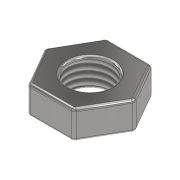
# Autodesk Inventor part: M3_nut
Saved by Autodesk Inventor 2020 (Build 240168000, 168)
## iProperties
Created: 2021-02-03
Part Number: M3_nut
Material: Generic
Document SubType Name: Modeling
Designer: JojoS
Density: 1 g/cm^3
Appearance: Steel - Polished
Author: JojoS
Autodesk Inventor part; units mm, degrees
ref_plane "YZ Plane" through (0, 0, 0) normal (1, 0, 0) x (0, 1, 0)
ref_plane "XZ Plane" through (0, 0, 0) normal (0, 1, 0) x (-1, 0, 0)
ref_plane "XY Plane" through (0, 0, 0) normal (0, 0, 1) x (1, 0, 0)
sketch "Sketch1" plane through (0, 0, 0) normal (0, 1, 0) x (-1, 0, 0)
  circle A0 centre (0, 0) radius 1.65
  line L0 (-1.7609, -3.05) -> (-3.5218, 0)
  line L1 (-3.5218, 0) -> (-1.7609, 3.05)
  line L2 (-1.7609, 3.05) -> (1.7609, 3.05)
  line L3 (1.7609, 3.05) -> (3.5218, 0)
  line L4 (3.5218, 0) -> (1.7609, -3.05)
  line L5 (1.7609, -3.05) -> (-1.7609, -3.05)
  dimension "d0" = 3.3
  dimension "d1" = 3.05
  constraints: 12 end point, 2 coincident, 1 centre point, 13 other
  measures "d0" diameter of A0
  measures "d1" distance from line of L5 point (0, 0)
extrude "Extrusion1" add sketch "Sketch1" along normal blind 2.2
fillet "Fillet1" radius 0.3 6 edges at (3.5218, 1.1, 0) (1.7609, 1.1, 3.05) (-1.7609, 1.1, 3.05) (-3.5218, 1.1, 0) (-1.7609, 1.1, -3.05) (1.7609, 1.1, -3.05)
thread "Thread1" size "M3x0.5" class "6H" standard "ANSI Metric M Profile" full length
fillet "Fillet2" radius 0.2 24 edges at (2.6414, 2.2, 1.525) (1.7377, 2.2, 3.0098) (0, 2.2, 3.05) (-1.7377, 2.2, 3.0098) (-2.6414, 2.2, 1.525) (-3.4754, 2.2, 0) (-2.6414, 2.2, -1.525) (-1.7377, 2.2, -3.0098) (0, 2.2, -3.05) (1.7377, 2.2, -3.0098) (2.6414, 2.2, -1.525) (3.4754, 2.2, 0) (2.6414, 0, -1.525) (1.7377, 0, -3.0098) (0, 0, -3.05) (-1.7377, 0, -3.0098) (-2.6414, 0, -1.525) (-3.4754, 0, 0) (-2.6414, 0, 1.525) (-1.7377, 0, 3.0098) (0, 0, 3.05) (1.7377, 0, 3.0098) (2.6414, 0, 1.525) (3.4754, 0, 0)
fillet "Fillet3" radius 0.2 2 edges at (1.65, 2.2, 0) (1.65, 0, 0)
body "Solid1"
